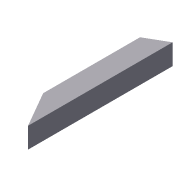
# Autodesk Inventor part: Frame_FrontAngle
Saved by Autodesk Inventor 2012 (Build 160160000, 160)
## iProperties
Created: 2012-01-09
Part Number: Frame_FrontAngle
Material: Aluminum-6061
Document SubType Name: Modeling
Designer: JesseK
Mass: 60.8399 g
Surface Area: 287.607 cm^2
Volume: 22.4501 cm^3
Density: 2.71 g/cm^3
Author: JesseK
Autodesk Inventor part; units mm, degrees
ref_plane "YZ Plane" through (0, 0, 0) normal (1, 0, 0) x (0, 1, 0)
ref_plane "XZ Plane" through (0, 0, 0) normal (0, 1, 0) x (-1, 0, 0)
ref_plane "XY Plane" through (0, 0, 0) normal (0, 0, 1) x (1, 0, 0)
sketch "Sketch1" plane through (0, 0, 0) normal (0, 0, 1) x (1, 0, 0)
  line L0 (0, 0) -> (25.4, 0)
  line L1 (25.4, 0) -> (25.4, 25.4)
  line L2 (25.4, 25.4) -> (0, 25.4)
  line L3 (0, 25.4) -> (0, 0)
  dimension "d0" = 25.4
  dimension "d1" = 25.4
  constraints: 8 end point, 2 parallel, 1 horizontal, 1 perpendicular
  measures "d0" distance of L1.end L2.end
  measures "d1" distance of L0.end L1.end
extrude "Extrusion1" add sketch "Sketch1" along normal blind 177.8
shell "Shell1" thickness 1.5875 removed faces 2 at (8.4667, 16.9333, 0) at (8.4667, 16.9333, 177.8)
sketch "Sketch2" plane through (0, 25.4, 0) normal (0, 1, 0) x (1, 0, 0)
  line L0 (0, -177.8) -> (25.4, -177.8) projected
  line L1 (25.4, 0) -> (0, 0) projected
  line L2 (0, 0) -> (0, -177.8) projected
  line L3 (0, 0) -> (0, -14.6647)
  line L4 (25.4, 0) -> (0, -14.6647)
  line L5 (0, 0) -> (25.4, 0)
  line L6 (0, -133.8059) -> (0, -177.8)
  line L7 (0, -177.8) -> (25.4, -177.8)
  line L8 (0, -133.8059) -> (25.4, -177.8)
  dimension "d5" = 60
  dimension "d6" = 30
  constraints: 12 end point, 2 perpendicular, 2 point on line, 1 collinear
  measures "d5" angle of L7 L8
  measures "d6" angle of L4 L1
extrude "Extrusion2" cut sketch "Sketch2" against normal through all
body "Solid1"
